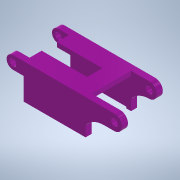
# Autodesk Inventor part: Dedo_2
Saved by Autodesk Inventor 2020 (Build 240168000, 168)
## iProperties
Created: 2021-07-29
Part Number: Dedo_2
Material: Generic
Document SubType Name: Modeling
Designer: chalo
Density: 1 g/cm^3
Appearance: Smooth - Purple
Author: chalo
Autodesk Inventor part; units mm, degrees
ref_plane "YZ Plane" through (0, 0, 0) normal (1, 0, 0) x (0, 1, 0)
ref_plane "XZ Plane" through (0, 0, 0) normal (0, 1, 0) x (-1, 0, 0)
ref_plane "XY Plane" through (0, 0, 0) normal (0, 0, 1) x (1, 0, 0)
sketch "Sketch1" plane through (0, 0, 0) normal (0, 0, 1) x (1, 0, 0)
  circle A0 centre (-22.3867, 3.2651) radius 1.1 projected
  circle A1 centre (-22.3867, 3.2651) radius 2.5
  line L0 (-22.3867, 5.7651) -> (-28.3867, 5.7651)
  arc A2 (-22.3867, 0.7651) -> (-28.3867, -2.2651) centre (-22.3867, -6.6901) ccw
  line L1 (-28.3867, -2.2651) -> (-28.3867, -5.7651)
  line L2 (-25.1757, -5.7651) -> (19.8243, -5.7651) construction
  line L3 (-28.3867, -5.7651) -> (-50.8867, -5.7651)
  line L4 (-28.3867, 5.7651) -> (-50.8867, 5.7651)
  line L5 (-50.8867, -5.7651) -> (-50.8867, 5.7651)
  point P0 (0, 0)
  dimension "d0" = 5
  dimension "d1" = 6
  dimension "d2" = 3.5
  dimension "d3" = 22.5
  constraints: 11 end point, 4 point on circle, 3 horizontal, 3 vertical alignment, 2 centre point, 2 tangent, 2 vertical, 1 coincident, 1 horizontal alignment
  measures "d0" diameter of A1
  measures "d1" distance of L0.start L0.end
  measures "d2" distance of L1.start L1.end
  measures "d3" distance of L1.end L3.end
extrude "Extrusion1" add sketch "Sketch1" along normal blind 2
sketch "Sketch2" plane through (0, 0, 0) normal (0, 0, -1) x (-1, 0, 0)
  line L0 (22.3867, 5.7651) -> (50.8867, 5.7651) projected
  arc A0 (22.3867, 5.7651) -> (22.3867, 0.7651) centre (22.3867, 3.2651) ccw projected
  arc A1 (28.3867, -2.2651) -> (22.3867, 0.7651) centre (22.3867, -6.6901) ccw projected
  line L1 (28.3867, -5.7651) -> (28.3867, -2.2651) projected
  line L2 (50.8867, -5.7651) -> (28.3867, -5.7651) projected
  line L3 (50.8867, 5.7651) -> (50.8867, -5.7651) projected
  circle A2 centre (22.3867, 3.2651) radius 1.1 projected
  line L4 (28.3867, -5.7651) -> (28.3867, -2.2651) projected
  line L5 (28.3867, -2.2651) -> (28.3867, 5.7651)
  point P0 (0, 0)
  constraints: 2 end point, 1 collinear, 1 point on line
extrude "Extrusion2" add sketch "Sketch2" along normal blind 15 contours L0 L3 L2 L1 L5
sketch "Sketch3" plane through (0, 0, -15) normal (0, 0, -1) x (-1, 0, 0)
  line L0 (28.3867, -5.7651) -> (50.8867, -5.7651) projected
  line L1 (50.8867, -5.7651) -> (50.8867, 5.7651) projected
  line L2 (50.8867, 5.7651) -> (28.3867, 5.7651) projected
  line L3 (28.3867, 5.7651) -> (28.3867, -5.7651) projected
  line L4 (28.3867, -2.2651) -> (28.3867, 5.7651) projected
  line L5 (22.3867, 5.7651) -> (28.3867, 5.7651) projected
  arc A0 (22.3867, 5.7651) -> (22.3867, 0.7651) centre (22.3867, 3.2651) ccw projected
  arc A1 (28.3867, -2.2651) -> (22.3867, 0.7651) centre (22.3867, -6.6901) ccw projected
  circle A2 centre (22.3867, 3.2651) radius 1.1 projected
  point P0 (0, 0)
extrude "Extrusion3" add sketch "Sketch3" against normal blind 2 contours A1 A0 L5 L3
sketch "Sketch4" plane through (0, 0, 2) normal (0, 0, 1) x (1, 0, 0)
  circle A0 centre (-18.8867, 3.2651) radius 1.1 projected
  line L0 (-22.3867, 5.7651) -> (-50.8867, 5.7651) projected
  line L1 (-50.8867, 5.7651) -> (-50.8867, -5.7651) projected
  line L2 (-50.8867, -5.7651) -> (-28.3867, -5.7651) projected
  line L3 (-28.3867, -5.7651) -> (-28.3867, -2.2651) projected
  arc A1 (-22.3867, 0.7651) -> (-28.3867, -2.2651) centre (-22.3867, -6.6901) ccw projected
  arc A2 (-22.3867, 0.7651) -> (-22.3867, 5.7651) centre (-22.3867, 3.2651) ccw projected
  circle A3 centre (-22.3867, 3.2651) radius 1.1 projected
  circle A4 centre (-18.8867, 3.2651) radius 2.5
  arc A5 (-22.3867, 0.7651) -> (-22.3867, 5.7651) centre (-22.3867, 3.2651) ccw projected
  line L4 (-22.3867, 5.7651) -> (-18.8867, 5.7651)
  line L5 (-22.3867, 0.7651) -> (-18.8867, 0.7651)
  point P0 (0, 0)
  point P1 (-19.9167, 3.6513)
  point P2 (-19.9167, 2.879)
  point P3 (-21.3567, 3.6513)
  point P4 (-21.3567, 2.879)
  dimension "d10" = 5
  constraints: 4 end point, 3 point on circle, 3 tangent, 1 centre point, 1 coincident, 1 parallel
  measures "d10" diameter of A4
extrude "Extrusion4" add sketch "Sketch4" against normal blind 2 contours A0 A2 A4 | A2 L4 A4 | A4 L5 A2 | A3 A4 picked at (-21.3511, 3.2651)
sketch "Sketch5" plane through (0, 0, 2) normal (0, 0, 1) x (1, 0, 0)
  arc A0 (-19.9167, 2.879) -> (-19.9167, 3.6513) centre (-22.3867, 3.2651) ccw projected
  arc A1 (-19.9167, 2.879) -> (-19.9167, 3.6513) centre (-18.8867, 3.2651) ccw projected
  line L0 (-22.3867, 0.7651) -> (-18.8867, 0.7651) projected
  arc A2 (-18.8867, 0.7651) -> (-18.8867, 5.7651) centre (-18.8867, 3.2651) ccw projected
  line L1 (-18.8867, 5.7651) -> (-50.8867, 5.7651) projected
  line L2 (-50.8867, 5.7651) -> (-50.8867, -5.7651) projected
  line L3 (-50.8867, -5.7651) -> (-28.3867, -5.7651) projected
  line L4 (-28.3867, -5.7651) -> (-28.3867, -2.2651) projected
  arc A3 (-22.3867, 0.7651) -> (-28.3867, -2.2651) centre (-22.3867, -6.6901) ccw projected
  arc A4 (-21.3567, 3.6513) -> (-21.3567, 2.879) centre (-22.3867, 3.2651) ccw projected
  arc A5 (-21.3567, 3.6513) -> (-21.3567, 2.879) centre (-18.8867, 3.2651) ccw projected
  circle A6 centre (-18.8867, 3.2651) radius 1.1
  point P0 (0, 0)
  constraints: 1 centre point, 1 coincident, 1 concentric
extrude "Extrusion5" add sketch "Sketch5" against normal blind 2 contours A5 A4
sketch "Sketch6" plane through (0, 0, 2) normal (0, 0, 1) x (1, 0, 0)
  arc A0 (-19.9167, 2.879) -> (-19.9167, 3.6513) centre (-18.8867, 3.2651) ccw projected
  circle A1 centre (-18.8867, 3.2651) radius 1.1
  point P0 (0, 0)
  constraints: 1 centre point, 1 coincident, 1 concentric
extrude "Extrusion6" cut sketch "Sketch6" against normal blind 2
shell "Shell1" thickness 1.5 removed faces 1 at (-43.3867, -5.7651, -9.3333)
sketch "Sketch7" plane through (0, 0, 2) normal (0, 0, 1) x (1, 0, 0)
  circle A0 centre (-18.8867, 3.2651) radius 1.1 projected
  line L0 (-22.3867, 0.7651) -> (-18.8867, 0.7651) projected
  arc A1 (-18.8867, 0.7651) -> (-18.8867, 5.7651) centre (-18.8867, 3.2651) ccw projected
  line L1 (-18.8867, 5.7651) -> (-50.8867, 5.7651) projected
  line L2 (-50.8867, 5.7651) -> (-50.8867, -5.7651) projected
  line L3 (-50.8867, -5.7651) -> (-28.3867, -5.7651) projected
  line L4 (-28.3867, -5.7651) -> (-28.3867, -2.2651) projected
  arc A2 (-22.3867, 0.7651) -> (-28.3867, -2.2651) centre (-22.3867, -6.6901) ccw projected
  line L5 (-50.8867, -5.7651) -> (-50.8867, 5.7651) projected
  line L6 (-50.8867, 5.7651) -> (-22.3867, 5.7651) projected
  circle A3 centre (-52.3867, 3.6651) radius 1.1
  line L7 (-53.3867, 4.7651) -> (-51.3867, 4.7651) construction
  circle A4 centre (-52.3867, 3.6651) radius 2.1
  line L8 (-50.8867, 5.7651) -> (-52.3867, 5.7651)
  line L9 (-52.3867, 1.5651) -> (-50.8867, 1.5651)
  point P0 (0, 0)
  point P1 (-52.3867, 4.7651)
  dimension "d19" = 2.2
  dimension "d20" = 1.5
  dimension "d21" = 2
  dimension "d23" = 1
  constraints: 6 end point, 3 horizontal, 3 tangent, 2 centre point, 2 point on circle, 1 coincident, 1 midpoint, 1 point on line, 1 vertical alignment
  measures "d19" diameter of A3
  measures "d20" distance from line of L2 A3.centre
  measures "d21" distance of L7.start L7.end
  measures "d23" distance between parallel lines of L6 L7
extrude "Extrusion7" add sketch "Sketch7" against normal blind 2 contours L2 A4 L8 | L9 A4 L2 | L2 A4 picked at (-51.02, 3.6651)
sketch "Sketch9" plane through (-50.8867, -5.7651, 2) normal (0, -1, 0) x (1, 0, 0)
  line L0 (1.5, -1.5) -> (21, -1.5) projected
  line L1 (21, -1.5) -> (21, -15.5) projected
  line L2 (21, -15.5) -> (1.5, -15.5) projected
  line L3 (1.5, -15.5) -> (1.5, -1.5) projected
  line L4 (22.5, -17) -> (22.5, 0) projected
  line L5 (0, 0) -> (22.5, 0) projected
  line L6 (0, -17) -> (0, 0) projected
  line L7 (22.5, -17) -> (0, -17) projected
  line L8 (-1.5, 0) -> (0, 0) projected
  line L9 (-1.5, 0) -> (-1.5, -2) projected
  line L10 (0, -2) -> (-1.5, -2) projected
  line L11 (0, 0) -> (0, -2) projected
  line L12 (0, -17) -> (0, -2) projected
  line L13 (0, -2) -> (1.5, -2)
  line L14 (21, -1.5) -> (21, -15.5) projected
  line L15 (21, -2) -> (22.5, -2)
  line L16 (0, -15) -> (1.5, -15)
  line L17 (1.5, -15.5) -> (1.5, -1.5) projected
  line L18 (21, -15) -> (22.5, -15)
  point P0 (50.8867, -2)
  dimension "d26" = 2
  constraints: 11 point on line, 8 end point, 1 horizontal, 1 perpendicular
  measures "d26" distance between parallel lines of L7 L16
extrude "Extrusion8" cut sketch "Sketch9" against normal up to surface (10.0303 mm away) contours L3 L16 L6 L13 | L15 L4 L18 L1
sketch "Sketch10" plane through (-50.8867, -5.7651, -15) normal (-1, 0, 0) x (0, 0, 1)
  line L0 (2, 10.0303) -> (15, 10.0303) projected
  line L1 (15, 10.0303) -> (15, 11.5303) projected
  line L2 (0, 11.5303) -> (15, 11.5303) projected
  line L3 (0, 0) -> (0, 11.5303) projected
  line L4 (0, 0) -> (2, 0) projected
  line L5 (2, 0) -> (2, 10.0303) projected
  line L6 (15, 7.3303) -> (15, 0) projected
  line L7 (15, 0) -> (17, 0) projected
  line L8 (17, 7.3303) -> (17, 0) projected
  line L9 (17, 7.3303) -> (15, 7.3303) projected
  point P0 (15, 5.7651)
extrude "Extrusion9" cut sketch "Sketch10" against normal blind 2
sketch "Sketch11" plane through (0, 0, -15) normal (0, 0, -1) x (-1, 0, 0)
  line L0 (48.8867, -5.7651) -> (48.8867, 5.7651) projected
  line L1 (48.8867, 5.7651) -> (22.3867, 5.7651) projected
  arc A0 (22.3867, 5.7651) -> (22.3867, 0.7651) centre (22.3867, 3.2651) ccw projected
  arc A1 (28.3867, -2.2651) -> (22.3867, 0.7651) centre (22.3867, -6.6901) ccw projected
  line L2 (28.3867, -2.2651) -> (28.3867, -5.7651) projected
  line L3 (28.3867, -5.7651) -> (48.8867, -5.7651) projected
  circle A2 centre (22.3867, 3.2651) radius 1.1 projected
  line L4 (48.8867, 1.5651) -> (49.3867, 1.5651) projected
  line L5 (49.3867, 4.2651) -> (49.3867, 1.5651) projected
  line L6 (29.8867, 4.2651) -> (49.3867, 4.2651) projected
  line L7 (29.8867, -5.7651) -> (29.8867, 4.2651) projected
  line L8 (48.8867, -5.7651) -> (29.8867, -5.7651) projected
  line L9 (48.8867, -5.7651) -> (48.8867, 1.5651) projected
  line L10 (49.3867, 1.5651) -> (52.3867, 1.5651) projected
  arc A3 (52.3867, 1.5651) -> (52.3867, 5.7651) centre (52.3867, 3.6651) ccw projected
  line L11 (52.3867, 5.7651) -> (48.8867, 5.7651) projected
  line L12 (48.8867, 5.7651) -> (48.8867, 4.2651) projected
  line L13 (49.3867, 4.2651) -> (48.8867, 4.2651) projected
  line L14 (49.3867, 1.5651) -> (49.3867, 4.2651) projected
  circle A4 centre (52.3867, 3.6651) radius 1.1 projected
  point P0 (0, 0)
extrude "Extrusion10" add sketch "Sketch11" against normal blind 2 contours L0 L6 L5 L4 | L0 L11 A3 L10 L5 L6
sketch "Sketch12" plane through (-28.3867, 5.7651, -13) normal (0, 1, 0) x (1, 0, 0)
  line L0 (-20.5, 0) -> (-20.5, -13) projected
  line L1 (-24, -13) -> (-20.5, -13) projected
  line L2 (-24, -15) -> (-24, -13) projected
  line L3 (9.5, -15) -> (-24, -15) projected
  line L4 (9.5, -15) -> (9.5, -13) projected
  line L5 (9.5, -13) -> (0, -13) projected
  line L6 (0, -13) -> (0, 0) projected
  line L7 (6, 0) -> (0, 0) projected
  line L8 (6, 2) -> (6, 0) projected
  line L9 (-24, 2) -> (6, 2) projected
  line L10 (-24, 2) -> (-24, 0) projected
  line L11 (-20.5, 0) -> (-24, 0) projected
  line L12 (-20.5, 0) -> (-20.5, -13) projected
  line L13 (-20.5, -2.5) -> (-5.5, -2.5)
  line L14 (-20.5, -10.5) -> (-5.5, -10.5)
  line L15 (-20.5, -6.5) -> (0, -6.5) construction
  line L16 (-5.5, -2.5) -> (-5.5, -10.5)
  point P0 (28.3867, -13)
  point P1 (-5.5, -6.5)
  dimension "d33" = 8
  dimension "d34" = 15
  constraints: 8 end point, 4 midpoint, 2 perpendicular, 2 point on line, 1 horizontal alignment, 1 vertical
  measures "d33" distance between parallel lines of L14 L13
  measures "d34" distance between parallel lines of L0 L16
extrude "Extrusion11" cut sketch "Sketch12" against normal blind 2 contours L13 L16 L14 L0
body "Solid1"
